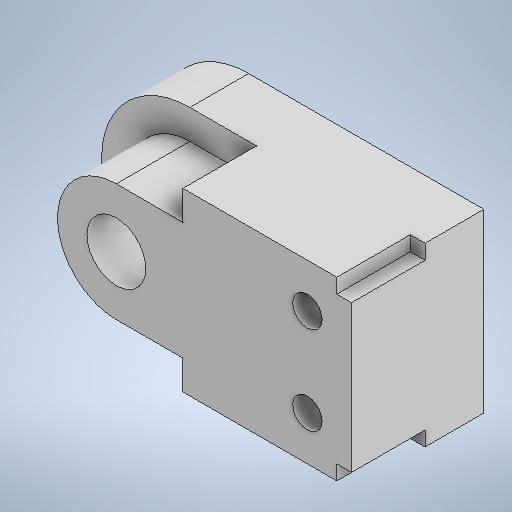
# Autodesk Inventor part: cad@31
Saved by Autodesk Inventor 2025.2 (Build 292293000, 293)
## iProperties
Created: 2025-03-17
Part Number: cad@31
Material: Generic
Document SubType Name: Modeling
Designer: spars
Density: 1 g/cm^3
Appearance: Default
Author: spars
Autodesk Inventor part; units mm, degrees
note: some values were not read from the file. Chosen so that the rebuilt part matches the saved one: direction of "Emboss1".
ref_plane "YZ Plane" through (0, 0, 0) normal (1, 0, 0) x (0, 1, 0)
ref_plane "XZ Plane" through (0, 0, 0) normal (0, 1, 0) x (-1, 0, 0)
ref_plane "XY Plane" through (0, 0, 0) normal (0, 0, 1) x (1, 0, 0)
sketch "Sketch1" plane through (0, 0, 0) normal (0, 0, 1) x (1, 0, 0)
  line L0 (-40, 30) -> (40, 30)
  line L1 (40, 30) -> (40, -30)
  line L2 (40, -30) -> (-40, -30)
  line L3 (-40, 30) -> (40, -30) construction
  line L4 (40, 30) -> (-40, -30) construction
  arc A0 (-40, 30) -> (-40, -30) centre (-40, 0) ccw
  point P0 (0, 0)
  dimension "d0" = 80
  dimension "d1" = 60
  constraints: 10 end point, 2 midpoint, 2 point on circle, 1 centre point, 1 horizontal, 1 parallel, 1 perpendicular
  measures "d0" distance of L1.end L2.end
  measures "d1" distance of L0.end L1.end
extrude "Extrusion1" add sketch "Sketch1" along normal blind 20
sketch "Sketch2" plane through (0, 0, 20) normal (0, 0, 1) x (1, 0, 0)
  line L0 (40, 30) -> (-40, 30) projected
  line L1 (-40, -30) -> (40, -30) projected
  arc A0 (-40, 20) -> (-40, -20) centre (-40, 0) ccw
  line L2 (-17.3383, 20) -> (-17.3383, 30)
  line L3 (-40, 20) -> (-17.3383, 20)
  line L4 (-17.3383, -20) -> (-17.3383, -30)
  line L5 (-40, -20) -> (-17.3383, -20)
  line L6 (-17.3383, 30) -> (35, 30)
  line L7 (35, 25) -> (40, 25)
  line L8 (35, -25) -> (40, -25)
  line L9 (40, -30) -> (40, 30) projected
  line L10 (-17.3383, 30) -> (35, 30)
  line L11 (-17.3383, -30) -> (35, -30)
  line L12 (35, 30) -> (35, 25)
  line L13 (35, -25) -> (35, -30)
  line L14 (40, 25) -> (40, -25)
  point P0 (0, 0)
  dimension "d4" = 20
  dimension "d6" = 5
  dimension "d8" = 5
  constraints: 24 end point, 8 point on line, 7 perpendicular, 3 collinear, 2 point on circle, 1 centre point, 1 horizontal
  measures "d4" radius of A0
  measures "d6" distance between parallel lines of L7 L6
  measures "d8" distance between parallel lines of L1 L8
extrude "Extrusion2" add sketch "Sketch2" along normal blind 25 contours L12 L7 L9 L8 L13 L1 L4 L5 A0 L3 L2 L0
sketch "Sketch3" plane through (0, 0, 45) normal (0, 0, 1) x (1, 0, 0)
  line L0 (-40, 20) -> (-17.3383, 20) projected
  circle A0 centre (-40, 0) radius 10
  circle A1 centre (25, 15) radius 5
  line L1 (35, 30) -> (-17.3383, 30) projected
  line L2 (0, 0) -> (38.2897, 0)
  line L3 (40, -25) -> (40, 25) projected
  circle A2 centre (25, -15) radius 5
  point P0 (-40, -20)
  dimension "d11" = 20
  dimension "d12" = 10
  dimension "d14" = 15
  dimension "d16" = 15
  constraints: 3 centre point, 2 end point, 1 horizontal, 1 symmetric about line, 1 other
  measures "d11" diameter of A0
  measures "d12" diameter of A1
  measures "d14" distance from line of L1 A1.centre
  measures "d16" distance from line of L3 A1.centre
extrude "Extrusion3" cut sketch "Sketch3" against normal through all
sketch "Sketch4" plane through (-40, -30, 0) normal (0, -1, 0) x (1, 0, 0)
  line L0 (37.6354, 35.5675) -> (61.1427, 35.5675) construction
  line L1 (61.1427, 35.5675) -> (61.1427, 25.3525) construction
  line L2 (61.1427, 25.3525) -> (37.6354, 25.3525) construction
  line L3 (37.6354, 25.3525) -> (37.6354, 35.5675) construction
  spline S0 degree 2 poles (41.3841, 25.3525) (40.3131, 25.3525) (38.8104, 25.8001) (38.147, 26.1198) knots 0 0 0 1 2 2 2
  line L4 (38.147, 26.1198) -> (38.147, 27.7664)
  line L5 (38.147, 27.7664) -> (38.2429, 27.7664)
  spline S1 degree 2 poles (38.2429, 27.7664) (38.8903, 27.1589) (40.5289, 26.4875) (41.2882, 26.4875) knots 0 0 0 1 2 2 2
  spline S2 degree 2 poles (41.2882, 26.4875) (42.3752, 26.4875) (43.4863, 27.3907) (43.4863, 28.1341) knots 0 0 0 1 2 2 2
  spline S3 degree 2 poles (43.4863, 28.1341) (43.4863, 28.7256) (42.9028, 29.4609) (42.2713, 29.6447) knots 0 0 0 1 2 2 2
  spline S4 degree 2 poles (42.2713, 29.6447) (41.8157, 29.7726) (41.0564, 29.9485) (40.4889, 30.0924) knots 0 0 0 1 2 2 2
  spline S5 degree 2 poles (40.4889, 30.0924) (39.9774, 30.2282) (39.1701, 30.6359) (38.8583, 30.9636) knots 0 0 0 1 2 2 2
  spline S6 degree 2 poles (38.8583, 30.9636) (38.5546, 31.2913) (38.2189, 32.1705) (38.2189, 32.746) knots 0 0 0 1 2 2 2
  spline S7 degree 2 poles (38.2189, 32.746) (38.2189, 33.945) (40.0893, 35.5675) (41.536, 35.5675) knots 0 0 0 1 2 2 2
  spline S8 degree 2 poles (41.536, 35.5675) (42.3673, 35.5675) (43.838, 35.2398) (44.4694, 34.9281) knots 0 0 0 1 2 2 2
  line L6 (44.4694, 34.9281) -> (44.4694, 33.3615)
  line L7 (44.4694, 33.3615) -> (44.3735, 33.3615)
  spline S9 degree 2 poles (44.3735, 33.3615) (43.9019, 33.7931) (42.4312, 34.4325) (41.6239, 34.4325) knots 0 0 0 1 2 2 2
  spline S10 degree 2 poles (41.6239, 34.4325) (40.7127, 34.4325) (39.5857, 33.5773) (39.5857, 32.8819) knots 0 0 0 1 2 2 2
  spline S11 degree 2 poles (39.5857, 32.8819) (39.5857, 32.2584) (40.2491, 31.5151) (40.8726, 31.3472) knots 0 0 0 1 2 2 2
  spline S12 degree 2 poles (40.8726, 31.3472) (41.2882, 31.2353) (42.4951, 30.9476) (42.8948, 30.8277) knots 0 0 0 1 2 2 2
  spline S13 degree 2 poles (42.8948, 30.8277) (43.9099, 30.516) (44.8531, 29.2611) (44.8531, 28.3419) knots 0 0 0 1 2 2 2
  spline S14 degree 2 poles (44.8531, 28.3419) (44.8531, 27.7584) (44.3815, 26.6394) (43.9579, 26.2477) knots 0 0 0 1 2 2 2
  spline S15 degree 2 poles (43.9579, 26.2477) (43.4863, 25.8161) (42.2873, 25.3525) (41.3841, 25.3525) knots 0 0 0 1 2 2 2
  line L8 (53.3816, 25.5284) -> (51.6791, 25.5284)
  line L9 (51.6791, 25.5284) -> (48.0742, 30.1163)
  line L10 (48.0742, 30.1163) -> (47.4987, 29.4689)
  line L11 (47.4987, 29.4689) -> (47.4987, 25.5284)
  line L12 (47.4987, 25.5284) -> (46.1879, 25.5284)
  line L13 (46.1879, 25.5284) -> (46.1879, 35.3917)
  line L14 (46.1879, 35.3917) -> (47.4987, 35.3917)
  line L15 (47.4987, 35.3917) -> (47.4987, 30.8597)
  line L16 (47.4987, 30.8597) -> (51.5432, 35.3917)
  line L17 (51.5432, 35.3917) -> (53.1418, 35.3917)
  line L18 (53.1418, 35.3917) -> (49.0574, 30.9876)
  line L19 (49.0574, 30.9876) -> (53.3816, 25.5284)
  line L20 (61.0708, 35.3917) -> (57.7377, 29.8925)
  line L21 (57.7377, 29.8925) -> (57.7377, 25.5284)
  line L22 (57.7377, 25.5284) -> (56.4269, 25.5284)
  line L23 (56.4269, 25.5284) -> (56.4269, 29.7566)
  line L24 (56.4269, 29.7566) -> (53.0938, 35.3917)
  line L25 (53.0938, 35.3917) -> (54.5485, 35.3917)
  line L26 (54.5485, 35.3917) -> (57.0903, 31.0515)
  line L27 (57.0903, 31.0515) -> (59.68, 35.3917)
  line L28 (59.68, 35.3917) -> (61.0708, 35.3917)
  point P0 (40, 0)
  constraints: 2 other
emboss "Emboss1" sketch "Sketch4" operation cut depth 2 direction (0, 1, 0)
body "Solid1"
